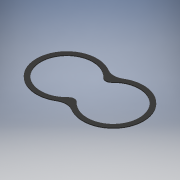
# Autodesk Inventor part: Dichtung
Saved by Autodesk Inventor 2017 (Build 210142000, 142)
## iProperties
Created: 2019-05-24
Part Number: Dichtung
Material: Rubber, Silicone
Document SubType Name: Modeling
Designer: Ole Simmering
Density: 1.25 g/cm^3
Appearance: Rubber - Black
Author: Ole Simmering
Autodesk Inventor part; units mm, degrees
ref_plane "YZ Plane" through (0, 0, 0) normal (1, 0, 0) x (0, 1, 0)
ref_plane "XZ Plane" through (0, 0, 0) normal (0, 1, 0) x (-1, 0, 0)
ref_plane "XY Plane" through (0, 0, 0) normal (0, 0, 1) x (1, 0, 0)
sketch "Sketch1" plane through (0, 0, 0) normal (0, 0, 1) x (1, 0, 0)
  line L0 (-11.999, -0.0009) -> (209.001, -0.0009) construction
  circle A0 centre (47.001, -0.0009) radius 42.5 construction
  circle A1 centre (132.001, -0.0009) radius 42.5 construction
  circle A2 centre (47.001, -0.0009) radius 47.5625 construction
  circle A3 centre (132.001, -0.0009) radius 47.5625 construction
  arc A4 (82.1177, 32.0773) -> (-0.5615, -0.0019) centre (47.001, -0.0009) ccw
  arc A5 (179.5635, -0.0009) -> (96.8843, 32.0773) centre (132.001, -0.0009) ccw
  arc A6 (-0.5615, -0.0019) -> (82.1177, -32.079) centre (47.001, -0.0009) ccw
  arc A7 (96.8843, -32.079) -> (179.5635, -0.0009) centre (132.001, -0.0009) ccw
  arc A8 (75.7238, 47.5616) -> (-8.5615, -0.0015) centre (47.001, -0.0009) ccw
  arc A9 (187.5635, -0.0009) -> (103.2782, 47.5616) centre (132.001, -0.0009) ccw
  line L1 (47.001, 47.5616) -> (132.001, 47.5616) construction
  arc A10 (75.7238, 47.5616) -> (103.2782, 47.5616) centre (89.501, 70.3754) ccw
  arc A11 (-8.5615, -0.0015) -> (75.7238, -47.5634) centre (47.001, -0.0009) ccw
  arc A12 (103.2782, -47.5634) -> (75.7238, -47.5634) centre (89.501, -70.3772) ccw
  arc A13 (103.2782, -47.5634) -> (187.5635, -0.0009) centre (132.001, -0.0009) ccw
  arc A14 (82.1177, 32.0773) -> (96.8843, 32.0773) centre (89.501, 38.8217) ccw
  line L2 (82.1177, 32.0773) -> (96.8843, 32.0773) construction
  arc A15 (96.8843, -32.079) -> (82.1177, -32.079) centre (89.501, -38.8234) ccw
  point P0 (0, 0)
  point P1 (89.501, 21.3519)
  point P2 (46.9513, 55.5616)
  point P3 (132.0501, 55.5616)
  dimension "d0" = 221
  dimension "d1" = 85
  dimension "d2" = 85
  dimension "d3" = 85
  dimension "d4" = 95.125
  dimension "d5" = 95.125
  dimension "d6" = 8
  dimension "d7" = 10
  constraints: 36 point on circle, 16 centre point, 6 end point, 6 symmetric about line, 5 point on line, 5 tangent, 3 horizontal, 2 coincident, 2 concentric, 7 other
  measures "d0" distance of L0.start L0.end
  measures "d1" diameter of A0
  measures "d2" diameter of A1
  measures "d3" distance of A1.centre A0.centre
  measures "d4" diameter of A2
  measures "d5" diameter of A3
  measures "d6" radial gap between concentric circles of A4 A8
  measures "d7" radius of A14
extrude "Extrusion1" add sketch "Sketch1" along normal blind 1.5
equation "\"d2\" = d1"
equation "\"d3\" = d1"
equation "\"d5\" = d4"
body "Solid1"
